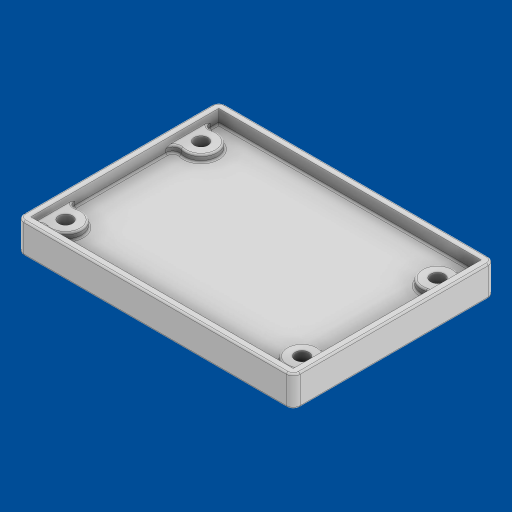
# Autodesk Inventor part: vma400_isolator
Saved by Autodesk Inventor 2023.2 (Build 272271000, 271)
## iProperties
Created: 2023-09-07
Part Number: vma400_isolator
Material: Generic
Document SubType Name: Modeling
Designer: agmlego
Density: 1 g/cm^3
Appearance: Default
Mass: 26.6409 g
Surface Area: 134.812 cm^2
Volume: 26.6409 cm^3
Author: agmlego
Autodesk Inventor part; units mm, degrees
ref_plane "YZ Plane" through (0, 0, 0) normal (1, 0, 0) x (0, 1, 0)
ref_plane "XZ Plane" through (0, 0, 0) normal (0, 1, 0) x (-1, 0, 0)
ref_plane "XY Plane" through (0, 0, 0) normal (0, 0, 1) x (1, 0, 0)
sketch "Sketch1" plane through (0, 0, 0) normal (0, 1, 0) x (-1, 0, 0)
  line L0 (38.5, 27.5) -> (-38.5, 27.5) construction
  line L1 (-38.5, 27.5) -> (-38.5, -27.5) construction
  line L2 (-38.5, -27.5) -> (38.5, -27.5) construction
  line L3 (38.5, -27.5) -> (38.5, 27.5) construction
  line L4 (38.5, 27.5) -> (-38.5, -27.5) construction
  line L5 (-38.5, 27.5) -> (38.5, -27.5) construction
  line L6 (34.9, 21.315) -> (-34.9, 21.315) construction
  line L7 (-34.9, 21.315) -> (-34.9, -18.685) construction
  line L8 (-34.9, -18.685) -> (34.9, -18.685) construction
  line L9 (34.9, -18.685) -> (34.9, 21.315) construction
  line L10 (34.9, 21.315) -> (-34.9, -18.685) construction
  line L11 (-34.9, 21.315) -> (34.9, -18.685) construction
  line L12 (0, 0) -> (0, 1.315) construction
  circle A0 centre (34.9, -18.685) radius 1.785 construction
  circle A1 centre (-34.9, -18.685) radius 1.785 construction
  circle A2 centre (-34.9, 21.315) radius 1.785 construction
  circle A3 centre (34.9, 21.315) radius 1.785 construction
  line L13 (38.75, -27.75) -> (-38.75, -27.75)
  line L14 (-38.75, -27.75) -> (-38.75, 27.75)
  line L15 (-38.75, 27.75) -> (38.75, 27.75)
  line L16 (38.75, 27.75) -> (38.75, -27.75)
  line L17 (-40.75, -29.75) -> (40.75, -29.75)
  line L18 (40.75, -29.75) -> (40.75, 29.75)
  line L19 (40.75, 29.75) -> (-40.75, 29.75)
  line L20 (-40.75, 29.75) -> (-40.75, -29.75)
  dimension "d0" = 77
  dimension "d1" = 55
  dimension "d2" = 69.8
  dimension "d3" = 40
  dimension "d4" = 3.57
  dimension "d5" = 4.4
  dimension "d6" = 0.25
  dimension "d7" = 2
  constraints: 42 end point, 8 coincident, 8 parallel, 4 centre point, 4 midpoint, 4 perpendicular, 3 equal radius, 2 horizontal, 1 vertical, 6 other
  measures "d0" distance of L2.end L1.end
  measures "d1" distance of L1.end L0.end
  measures "d2" distance of L8.end L7.end
  measures "d3" distance of L7.end L6.end
  measures "d4" diameter of A0
  measures "d5" distance edge to line of A3 L0
  measures "d6" distance between parallel lines of L2 L13
  measures "d7" distance between parallel lines of L13 L17
extrude "Extrusion1" add sketch "Sketch1" along normal blind 4
extrude "Extrusion2" add sketch "Sketch1" against normal blind 5 contours L13 L14 L15 L16 | L20 L19 L18 L17
sketch "Sketch2" plane through (0, 0, 0) normal (0, 1, 0) x (1, 0, 0)
  circle A0 centre (-34.9, -21.315) radius 1.785 construction
  circle A1 centre (-34.9, 18.685) radius 1.785 construction
  circle A2 centre (34.9, 18.685) radius 1.785 construction
  circle A3 centre (34.9, -21.315) radius 1.785 construction
  circle A4 centre (34.9, -21.315) radius 4.785
  circle A5 centre (34.9, 18.685) radius 4.785
  circle A6 centre (-34.9, 18.685) radius 4.785
  circle A7 centre (-34.9, -21.315) radius 4.785
  point P0 (0, 0)
  dimension "d12" = 3
  dimension "d13" = 3
  dimension "d14" = 3
  dimension "d15" = 3
  constraints: 4 centre point
  measures "d12" radial gap between concentric circles of A3 A4
  measures "d13" radial gap between concentric circles of A2 A5
  measures "d14" radial gap between concentric circles of A1 A6
  measures "d15" radial gap between concentric circles of A0 A7
extrude "Extrusion3" add sketch "Sketch2" along normal blind 2
hole "Hole1" at (-34.9, 0, -18.685) at (34.9, 0, -18.685) at (34.9, 0, 21.315) at (-34.9, 0, 21.315) direction (0, -1, 0) diameter 4.0386 depth 4.5 start extended yes
fillet "Fillet1" radius 2 8 edges at (-38.75, 1, 18.4736) (-38.75, 1, 24.1564) (-38.75, 1, -15.8436) (-38.75, 1, -21.5264) (38.75, 1, -15.8436) (38.75, 1, -21.5264) (38.75, 1, 18.4736) (38.75, 1, 24.1564)
fillet "Fillet2" radius 2 4 edges at (-40.75, -0.5, 29.75) (-40.75, -0.5, -29.75) (40.75, -0.5, -29.75) (40.75, -0.5, 29.75)
fillet "Fillet3" radius 0.5 48 edges at (40.1642, 4, 29.1642) (40.75, 4, 0) (40.1642, 4, -29.1642) (0, 4, -29.75) (-40.1642, 4, -29.1642) (-40.75, 4, 0) (-40.1642, 4, 29.1642) (0, 4, 29.75) (-40.1642, -5, 29.1642) (-40.75, -5, 0) (-40.1642, -5, -29.1642) (0, -5, -29.75) (40.1642, -5, -29.1642) (40.75, -5, 0) (40.1642, -5, 29.1642) (0, -5, 29.75) (37.9561, 0, -23.6175) (38.75, 0, -26.4815) (37.9561, 0, -13.7525) (38.75, 0, 1.315) (37.9561, 0, 16.3825) (30.115, 0, 21.315) (37.9187, 0, 26.2199) (30.115, 0, -18.685) (0, 0, -27.75) (37.9561, 2, -13.7525) (37.9561, 2, -23.6175) (30.115, 2, -18.685) (38.7489, 2, 27.75) (37.9187, 2, 26.2199) (37.9561, 2, 16.3825) (30.115, 2, 21.315) (0, 0, 27.75) (-37.9561, 2, 16.3825) (-38.7489, 2, 27.75) (-37.9187, 2, 26.2199) (-30.115, 2, 21.315) (-37.9187, 0, 26.2199) (-37.9561, 0, 16.3825) (-38.75, 0, 1.315) (-37.9561, 0, -13.7525) (-30.115, 0, -18.685) (-37.9561, 0, -23.6175) (-38.75, 0, -26.4815) (-30.115, 0, 21.315) (-30.115, 2, -18.685) (-37.9561, 2, -23.6175) (-37.9561, 2, -13.7525)
body "Solid1"
